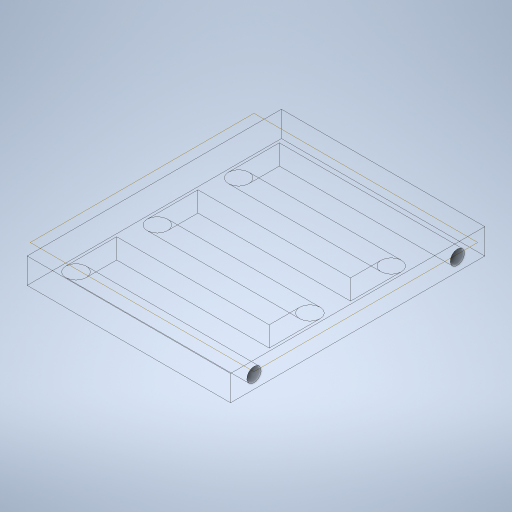
# Autodesk Inventor part: strain gauge v2
Saved by Autodesk Inventor 2024.2 (Build 282272000, 272)
## iProperties
Created: 2024-07-11
Part Number: strain gauge v2
Material: Generic
Document SubType Name: Modeling
Designer: Tom
Density: 1 g/cm^3
Appearance: Default
Author: Tom
Autodesk Inventor part; units mm, degrees
ref_plane "YZ Plane" through (0, 0, 0) normal (1, 0, 0) x (0, 1, 0)
ref_plane "XY Plane" through (0, 0, 0) normal (0, 0, 1) x (1, 0, 0)
ref_plane "Work Plane1" through (0, 1.5875, 0) normal (0, 1, 0) x (-1, 0, 0)
sketch "Sketch8" plane through (0, 0, 0) normal (0, 1, 0) x (-1, 0, 0)
  line L0 (0, 0) -> (22.225, 0)
  line L1 (22.225, 0) -> (22.225, -5.08)
  line L2 (22.225, -5.08) -> (3.175, -5.08)
  line L3 (3.175, -5.08) -> (3.175, -10.16)
  line L4 (3.175, -10.16) -> (22.225, -10.16)
  line L5 (22.225, -10.16) -> (22.225, -15.2317)
  line L6 (22.225, -15.2317) -> (3.175, -15.2317)
  line L7 (3.175, -15.2317) -> (3.175, -20.3117)
  line L8 (3.175, -20.3117) -> (22.225, -20.3117)
  line L9 (22.225, -20.3117) -> (22.225, -25.393)
  line L10 (22.225, -25.393) -> (0, -25.393)
  dimension "d24" = 22.225
  dimension "d25" = 5.08
  dimension "d26" = 19.05
  dimension "d27" = 5.08
  dimension "d28" = 5.08
  constraints: 22 end point, 5 perpendicular, 4 horizontal, 2 vertical
  measures "d24" distance of L0.start L0.end
  measures "d25" distance of L0.end L1.end
  measures "d26" distance of L1.end L2.end
  measures "d27" distance of L2.end L3.end
  measures "d28" distance of L6.end L7.end
sketch "Sketch9" plane through (0, 0, 0) normal (1, 0, 0) x (0, 1, 0)
  circle A0 centre (0, 0) radius 0.889
  dimension "d29" = 1.778
  constraints: 1 centre point, 1 coincident
  measures "d29" diameter of A0
sketch "Sketch10" plane through (0, 1.5875, 0) normal (0, 1, 0) x (-1, 0, 0)
  line L0 (0, 2.9232) -> (25.4, 2.9232)
  line L1 (25.4, 2.9232) -> (25.4, -28.8268)
  line L2 (25.4, -28.8268) -> (0, -28.8268)
  line L3 (0, -28.8268) -> (0, 2.9232)
  point P0 (0, 0)
  dimension "d30" = 25.4
  dimension "d32" = 31.75
  constraints: 8 end point, 2 parallel, 1 horizontal, 1 perpendicular
  measures "d30" distance of L0.start L0.end
  measures "d32" distance of L2.end L0.start
extrude "Extrusion4" add sketch "Sketch10" against normal blind 3.175
sweep "Sweep2" cut profiles "Sketch9" path "Sketch8"
body "Solid2"
